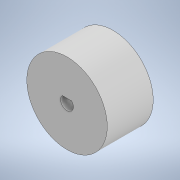
# Autodesk Inventor part: felga
Saved by Autodesk Inventor 2020.3 (Build 243373000, 373)
## iProperties
Created: 2021-03-19
Part Number: felga
Material: Ogólny
Document SubType Name: Modeling
Designer: patry
Density: 1 g/cm^3
Appearance: Domyślna
Author: patry
Autodesk Inventor part; units mm, degrees
ref_plane "YZ Plane" through (0, 0, 0) normal (1, 0, 0) x (0, 1, 0)
ref_plane "XZ Plane" through (0, 0, 0) normal (0, 1, 0) x (-1, 0, 0)
ref_plane "XY Plane" through (0, 0, 0) normal (0, 0, 1) x (1, 0, 0)
sketch "Szkic1" plane through (0, 0, 0) normal (0, 0, 1) x (1, 0, 0)
  line L0 (2.3165, 0) -> (0.0582, 0) construction
  arc A0 (1.1874, -2.3597) -> (2.3165, 0) centre (1.1874, -0.9097) ccw construction
  arc A1 (0.0582, 0) -> (1.1874, -2.3597) centre (1.1874, -0.9097) ccw construction
  circle A2 centre (1.1874, -0.9097) radius 10.5
  line L1 (-0.0447, 0.225) -> (2.4195, 0.225)
  arc A3 (2.8624, -0.9097) -> (2.4195, 0.225) centre (1.1874, -0.9097) ccw
  arc A4 (-0.0447, 0.225) -> (2.8624, -0.9097) centre (1.1874, -0.9097) ccw
  circle A5 centre (1.1874, -0.9097) radius 8.5
  point P0 (0, 0)
  dimension "d0" = 21
  dimension "d7" = 1.45
  dimension "d8" = 0.225
  dimension "d9" = 17
  constraints: 8 point on circle, 6 centre point, 4 end point, 2 coincident, 2 other
  measures "d0" diameter of A2
  measures "d7" radius of A0
  measures "d8" distance between parallel lines of L0 L1
  measures "d9" diameter of A5
extrude "Wyciągnięcie proste1" add sketch "Szkic1" along normal blind 7 contours A2 | A5
sketch "Szkic3" plane through (1.1874, -0.9097, 0) normal (0, 0, -1) x (-1, 0, 0)
  point P0 (1.1874, 0.9097)
extrude "Wyciągnięcie proste3" add sketch "Szkic1" against normal blind 5 contours A2
